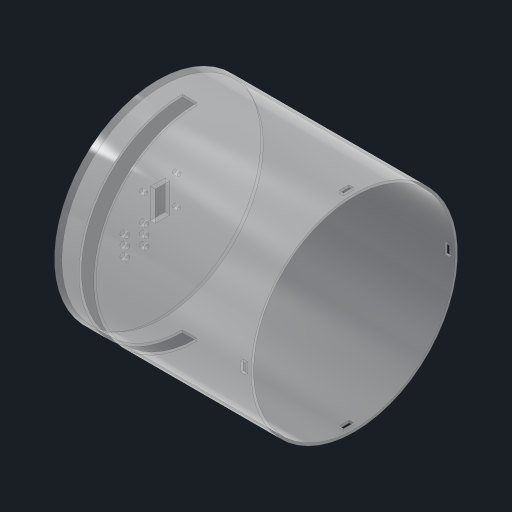
# Autodesk Inventor part: OUTK_001_ChipBucket
Saved by Autodesk Inventor 2024.2 (Build 282272000, 272)
## iProperties
Created: 2024-11-24
Part Number: OUTK_001_ChipBucket
Material: Polycarbonate, Clear
Document SubType Name: Modeling
Designer: Bryan
Density: 1.2 g/cm^3
Appearance: Polycarbonate - Clear
Mass: 1168.4 g
Surface Area: 5137.97 cm^2
Volume: 973.669 cm^3
Author: Bryan
Autodesk Inventor part; units mm, degrees
ref_plane "YZ Plane" through (0, 0, 0) normal (1, 0, 0) x (0, 1, 0)
ref_plane "XZ Plane" through (0, 0, 0) normal (0, 1, 0) x (-1, 0, 0)
ref_plane "XY Plane" through (0, 0, 0) normal (0, 0, 1) x (1, 0, 0)
sketch "Sketch1" plane through (0, 0, 0) normal (1, 0, 0) x (0, 1, 0)
  circle A0 centre (0, 0) radius 133.35
  dimension "d0" = 266.7
  constraints: 1 centre point, 1 coincident
  measures "d0" diameter of A0
extrude "Extrusion1" add sketch "Sketch1" along normal mid plane 254
sketch "Sketch2" plane through (127, 0, 0) normal (1, 0, 0) x (0, 0, -1)
  circle A0 centre (0, 0) radius 130.175
  dimension "d3" = 260.35
  constraints: 1 centre point, 1 coincident
  measures "d3" diameter of A0
extrude "Extrusion2" cut sketch "Sketch2" against normal blind 247.65
sketch "Sketch3" plane through (0, 0, 0) normal (0, 0, 1) x (1, 0, 0)
  line L0 (127, 130.175) -> (127, -130.175) projected
  line L1 (127, 130.175) -> (-120.65, 130.175) projected
  line L2 (127, -130.175) -> (-120.65, -130.175) projected
  line L3 (-95.25, 130.175) -> (-95.25, -130.175)
  line L4 (-76.2, -130.175) -> (-76.2, 130.175)
  line L5 (-120.65, 130.175) -> (-120.65, -130.175) projected
  point P0 (0, 0)
  point P1 (-139.7, 130.175)
  point P2 (-139.7, -130.175)
  dimension "d7" = 19.05
  dimension "d61" = 25.4
  constraints: 4 end point, 4 point on line, 1 parallel, 1 vertical
  measures "d7" distance between parallel lines of L3 L4
  measures "d61" distance between parallel lines of L3 L5
extrude "Extrusion3" cut sketch "Sketch3" along normal blind 266.7 contours L4 L2 L3 L1
sketch "Sketch4" plane through (0, 0, 0) normal (0, 1, 0) x (-1, 0, 0)
  line L0 (95.25, 0) -> (76.2, 0) projected
  line L1 (95.25, 0) -> (95.25, 28.9256) projected
  line L2 (76.2, 0) -> (76.2, 28.9256) projected
  line L3 (76.2, 28.9256) -> (95.25, 28.9256) projected
  point P0 (0, 0)
extrude "Extrusion4" cut sketch "Sketch4" along normal through all both and the other way through all
sketch "Sketch5" plane through (0, 0, 0) normal (0, 1, 0) x (-1, 0, 0)
  line L0 (-113.665, 6.35) -> (-119.38, 6.35)
  line L1 (-119.38, 6.35) -> (-119.38, -6.35)
  line L2 (-119.38, -6.35) -> (-113.665, -6.35)
  line L3 (-113.665, -6.35) -> (-113.665, 6.35)
  line L4 (-127, 133.35) -> (-127, -133.35) projected
  point P0 (0, 0)
  point P1 (-113.665, 0)
  dimension "d12" = 5.715
  dimension "d13" = 12.7
  dimension "d14" = 7.62
  constraints: 8 end point, 2 parallel, 1 horizontal, 1 horizontal alignment, 1 midpoint, 1 perpendicular
  measures "d12" distance of L2.end L1.end
  measures "d13" distance of L1.end L0.end
  measures "d14" distance between parallel lines of L4 L1
extrude "Extrusion5" cut sketch "Sketch5" along normal through all both and the other way through all
sketch "Sketch6" plane through (0, 0, 0) normal (0, 0, 1) x (1, 0, 0)
  line L0 (113.665, 6.35) -> (119.38, 6.35)
  line L1 (119.38, 6.35) -> (119.38, -6.35)
  line L2 (119.38, -6.35) -> (113.665, -6.35)
  line L3 (113.665, -6.35) -> (113.665, 6.35)
  line L4 (127, -133.35) -> (127, 133.35) projected
  point P0 (0, 0)
  point P1 (113.665, 0)
  dimension "d17" = 5.715
  dimension "d18" = 12.7
  dimension "d19" = 7.62
  constraints: 8 end point, 2 parallel, 1 horizontal, 1 horizontal alignment, 1 midpoint, 1 perpendicular
  measures "d17" distance of L1.end L2.end
  measures "d18" distance of L0.end L1.end
  measures "d19" distance between parallel lines of L4 L1
extrude "Extrusion6" cut sketch "Sketch6" along normal through all both and the other way through all
sketch "Sketch8" plane through (-127, 0, 0) normal (-1, 0, 0) x (0, 0, 1)
  line L0 (-9.525, -19.05) -> (9.525, -19.05)
  line L1 (9.525, -19.05) -> (9.525, 19.05)
  line L2 (9.525, 19.05) -> (-9.525, 19.05)
  line L3 (-9.525, 19.05) -> (-9.525, -19.05)
  circle A0 centre (20.6375, -14.7172) radius 3.2512
  circle A1 centre (20.6375, -40.1172) radius 3.2512
  circle A2 centre (45.5295, -14.7172) radius 3.2512
  circle A3 centre (45.5295, -40.1172) radius 3.2512
  line L4 (-9.525, -14.4526) -> (9.525, -14.4526) construction
  line L5 (0, -14.4526) -> (0, -40.3818) construction
  line L6 (20.6375, -14.7172) -> (20.6375, -40.1172) construction
  line L7 (-6.35, -16.6687) -> (-6.35, 15.875) construction
  line L8 (-6.35, 15.875) -> (6.35, 15.875) construction
  line L9 (6.35, 15.875) -> (6.35, -16.6687) construction
  line L10 (6.35, -16.6687) -> (-6.35, -16.6687) construction
  line L11 (-6.35, -8.8963) -> (-2.3812, -4.9276) construction
  line L12 (-2.3812, -4.9276) -> (-2.3812, 7.7724) construction
  line L13 (6.35, 11.7412) -> (2.3813, 7.7724) construction
  line L14 (2.3813, 7.7724) -> (2.3813, -4.9276) construction
  line L15 (2.3813, -4.9276) -> (6.35, -8.8963) construction
  line L16 (0, -16.6687) -> (0, 15.875) construction
  line L17 (-2.3812, 7.7724) -> (-6.35, 11.7412) construction
  line L18 (2.3813, 7.7724) -> (21.4312, 7.7724) construction
  line L19 (21.4312, 7.7724) -> (21.4312, -4.9276) construction
  line L20 (21.4312, -4.9276) -> (2.3813, -4.9276) construction
  line L21 (2.3813, -4.9276) -> (2.3813, 7.7724) construction
  line L22 (-2.3812, 7.7724) -> (-21.4312, 7.7724) construction
  line L23 (-21.4312, 7.7724) -> (-21.4312, -4.9276) construction
  line L24 (-21.4312, -4.9276) -> (-2.3812, -4.9276) construction
  line L25 (-2.3812, -4.9276) -> (-2.3812, 7.7724) construction
  line L26 (-15.0812, 14.1224) -> (-8.7312, 14.1224) construction
  line L27 (-8.7312, 14.1224) -> (-8.7312, -11.2776) construction
  line L28 (-8.7312, -11.2776) -> (-15.0812, -11.2776) construction
  line L29 (-15.0812, -11.2776) -> (-15.0812, 14.1224) construction
  line L30 (-21.4312, 1.4224) -> (-15.0812, 1.4224) construction
  circle A4 centre (-21.4312, -17.6276) radius 2.4892
  circle A5 centre (-21.4312, 20.4724) radius 2.4892
  circle A6 centre (21.4312, 20.4724) radius 2.4892
  line L31 (-6.35, -19.05) -> (6.35, -19.05)
  line L32 (6.35, -19.05) -> (6.35, -43.5568) construction
  line L33 (6.35, -43.5568) -> (-6.35, -43.5568) construction
  line L34 (-6.35, -43.5568) -> (-6.35, -19.05) construction
  circle A7 centre (20.6375, -27.4172) radius 3.2512
  circle A8 centre (45.5295, -27.4172) radius 3.2512
  line L35 (7.1437, -11.2776) -> (16.6688, -11.2776) construction
  line L36 (16.6688, -11.2776) -> (16.6688, -4.9276) construction
  line L37 (16.6688, -4.9276) -> (7.1437, -4.9276) construction
  line L38 (7.1437, -4.9276) -> (7.1437, -11.2776) construction
  point P0 (0, 0)
  point P1 (0, -27.4172)
  point P2 (-2.3812, 1.4224)
  point P3 (0, -0.3969)
  point P4 (0, 19.05)
  point P5 (-9.525, 0)
  point P6 (-11.9062, 14.1224)
  point P7 (-11.9062, 7.7724)
  point P8 (-11.9062, -11.2776)
  point P9 (-18.2562, 1.4224)
  point P10 (0, -43.5568)
  point P11 (0, -19.05)
  point P12 (11.9062, -4.9276)
  point P13 (11.9062, 7.7724)
  dimension "d22" = 19.05
  dimension "d23" = 38.1
  dimension "d24" = 6.5024
  dimension "d25" = 25.4
  dimension "d26" = 24.892
  dimension "d28" = 11.1125
  dimension "d31" = 4.5974
  dimension "d32" = 25.9292
  dimension "d35" = 3.175
  dimension "d36" = 3.175
  dimension "d37" = 3.175
  dimension "d38" = 2.3813
  dimension "d39" = 3.9688
  dimension "d40" = 12.7
  dimension "d41" = 45
  dimension "d42" = 45
  dimension "d44" = 19.05
  dimension "d45" = 6.35
  dimension "d46" = 25.4
  dimension "d47" = 7.7724
  dimension "d56" = 12.7
  dimension "d57" = 4.9784
  dimension "d62" = 12.7
  dimension "d63" = 3.175
  dimension "d64" = 9.525
  dimension "d65" = 6.35
  constraints: 78 end point, 19 midpoint, 12 parallel, 10 horizontal, 9 centre point, 8 horizontal alignment, 8 vertical alignment, 7 point on line, 6 equal length, 6 perpendicular, 6 vertical, 5 equal radius, 1 coincident, 1 collinear, 1 symmetric about line, 2 other
  measures "d22" distance of L2.end L1.end
  measures "d23" distance of L1.end L0.end
  measures "d24" diameter of A0
  measures "d25" distance of A3.centre A2.centre
  measures "d26" distance of A3.centre L6.end
  measures "d28" distance from line of L6.end L1
  measures "d31" distance between parallel lines of L0 L4
  measures "d32" distance of L5.start L5.end
  measures "d35" distance between parallel lines of L2 L8
  measures "d36" distance between parallel lines of L3 L7
  measures "d37" distance between parallel lines of L1 L9
  measures "d38" distance between parallel lines of L0 L10
  measures "d39" distance between parallel lines of L9 L14
  measures "d40" distance of L13.end L14.end
  measures "d41" angle of L11 L7
  measures "d42" angle of L7 L17
  measures "d44" distance of L12.end L22.end
  measures "d45" distance of L27.end L28.end
  measures "d46" distance of L28.end L26.start
  measures "d47" distance from line of L10 L15.end
  measures "d56" distance of A4.centre L23.end
  measures "d57" diameter of A4
  measures "d62" distance of L32.end L33.end
  measures "d63" distance from line of L5.end L33
  measures "d64" distance of L37.end L36.end
  measures "d65" distance of L36.end L35.end
extrude "Extrusion7" cut sketch "Sketch8" against normal blind 25.4
body "Solid1"
